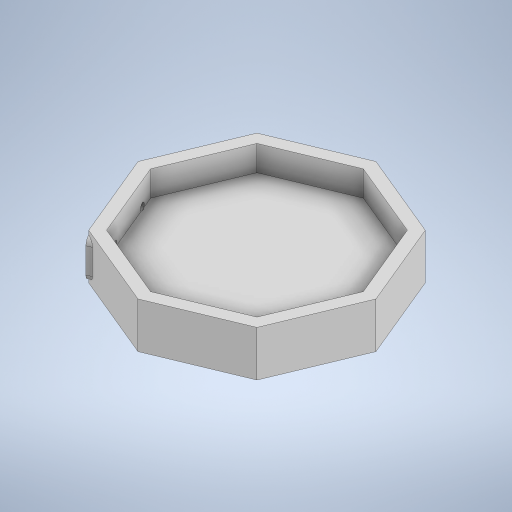
# Autodesk Inventor part: base1
Saved by Autodesk Inventor 2023 (Build 270158000, 158)
## iProperties
Created: 2025-10-17
Part Number: base1
Material: Generic
Document SubType Name: Modeling
Designer: Justin Pascual
Density: 1 g/cm^3
Appearance: Default
Author: Justin Pascual
Autodesk Inventor part; units mm, degrees
ref_plane "XZ Plane" through (0, 0, 0) normal (0, 1, 0) x (-1, 0, 0)
ref_plane "XY Plane" through (0, 0, 0) normal (0, 0, 1) x (1, 0, 0)
ref_plane "Work Plane2" through (0, 0, 0) normal (0.9238795, 0, -0.3826834) x (0, 1, 0)
sketch "Sketch1" plane through (0, 0, 0) normal (0, 1, 0) x (-1, 0, 0)
  line L0 (0, 0) -> (-59.69, 0) construction
  line L1 (-59.69, 0) -> (-42.2072, 42.2072)
  line L2 (-42.2072, 42.2072) -> (0, 59.69)
  line L3 (0, 59.69) -> (42.2072, 42.2072)
  line L4 (42.2072, 42.2072) -> (59.69, 0)
  line L5 (59.69, 0) -> (42.2072, -42.2072)
  line L6 (42.2072, -42.2072) -> (0, -59.69)
  line L7 (0, -59.69) -> (-42.2072, -42.2072)
  line L8 (-42.2072, -42.2072) -> (-59.69, 0)
  dimension "d0" = 59.69
  constraints: 18 end point, 1 coincident, 1 horizontal, 17 other
  measures "d0" distance of L0.start L0.end
extrude "Extrusion1" add sketch "Sketch1" along normal blind 22.86
sketch "Sketch2" plane through (0, 22.86, 0) normal (0, 1, 0) x (1, 0, 0)
  line L0 (0, 0) -> (53.34, 0) construction
  line L1 (53.34, 0) -> (37.7171, -37.7171)
  line L2 (37.7171, -37.7171) -> (0, -53.34)
  line L3 (0, -53.34) -> (-37.7171, -37.7171)
  line L4 (-37.7171, -37.7171) -> (-53.34, 0)
  line L5 (-53.34, 0) -> (-37.7171, 37.7171)
  line L6 (-37.7171, 37.7171) -> (0, 53.34)
  line L7 (0, 53.34) -> (37.7171, 37.7171)
  line L8 (37.7171, 37.7171) -> (53.34, 0)
  dimension "d3" = 53.34
  constraints: 18 end point, 2 coincident, 1 horizontal, 17 other
  measures "d3" distance of L0.start L0.end
ref_plane "Work Plane3" through (13.2151, 0, -64.0151) normal (0.7071068, 0, -0.7071068) x (-0.7071068, 0, -0.7071068)
sketch "Sketch8" plane through (-33.0485, -8.2404, -79.7862) normal (0.9238795, 0, -0.3826834) x (0.3826834, 0, 0.9238795)
  line L0 (108.585, -29.1954) -> (64.135, -29.1954)
  line L1 (60.96, -26.0204) -> (60.96, -13.3204)
  line L2 (64.135, -10.1454) -> (108.585, -10.1454)
  line L3 (111.76, -13.3204) -> (111.76, -26.0204)
  arc A0 (108.585, -29.1954) -> (111.76, -26.0204) centre (108.585, -26.0204) ccw
  arc A1 (111.76, -13.3204) -> (108.585, -10.1454) centre (108.585, -13.3204) ccw
  arc A2 (64.135, -10.1454) -> (60.96, -13.3204) centre (64.135, -13.3204) ccw
  arc A3 (60.96, -26.0204) -> (64.135, -29.1954) centre (64.135, -26.0204) ccw
  line L4 (109.2024, -31.1004) -> (63.5176, -31.1004) projected
  line L5 (86.36, 17.6501) -> (86.36, -39.2254) projected
  point P0 (0, 0)
  point P1 (111.76, -29.1954)
  point P2 (60.96, -10.1454)
  point P3 (111.76, -10.1454)
  dimension "d43" = 19.05
  dimension "d42" = 50.8
  dimension "d39" = 3.175
  dimension "d47" = 1.905
  dimension "d48" = 25.4
  dimension "d49" = 25.4
  constraints: 8 end point, 8 point on circle, 8 tangent, 6 point on line, 4 centre point, 3 equal radius, 2 parallel, 1 horizontal, 1 perpendicular
  measures "d43" distance of point (111.76, -10.145) point (111.76, -29.195)
  measures "d42" distance of point (60.96, -10.145) point (111.76, -10.145)
  measures "d39" radius of A0
  measures "d47" distance between parallel lines of L4 L0
  measures "d48" distance between parallel lines of L5 L1
  measures "d49" distance between parallel lines of L5 L3
extrude "Extrusion5" add sketch "Sketch8" against normal up to surface (55.1464 mm away)
extrude "Extrusion4" cut sketch "Sketch2" against normal blind 12.7
sketch "Sketch9" plane through (-41.2284, 5.08, 44.5701) normal (-0.9238795, 0, 0.3826834) x (0.3826834, 0, 0.9238795)
  line L0 (0, 12.7) -> (0, 0) projected
  line L1 (-50.8, 0) -> (-50.8, 12.7) projected
  line L2 (-48.2424, -5.08) -> (-2.5576, -5.08) projected
  point P0 (-25.4, -5.08)
  point P1 (-38.1, 6.35)
  point P2 (-12.7, 6.35)
  dimension "d50" = 25.4
  dimension "d51" = 12.7
  dimension "d52" = 12.7
  dimension "d53" = 11.43
  measures "d50" distance of point (-38.1, 6.35) point (-12.7, 6.35)
  measures "d51" distance from line of L0 point (-12.7, 6.35)
  measures "d52" distance from line of L1 point (-38.1, 6.35)
  measures "d53" distance from line of L2 point (-38.1, 6.35)
hole "Hole2" at (-55.8087, 11.43, 9.3703) at (-46.0885, 11.43, 32.8369) direction (0.9238795, 0, -0.3826834) diameter 3.4544 depth 5.8666 tip angle 118 clearance for "Flat Head Machine Screw (82)" size "#5" standard "Ansi Unified Screw Threads"
equation "\"d48\" = d49"
body "Solid1"
